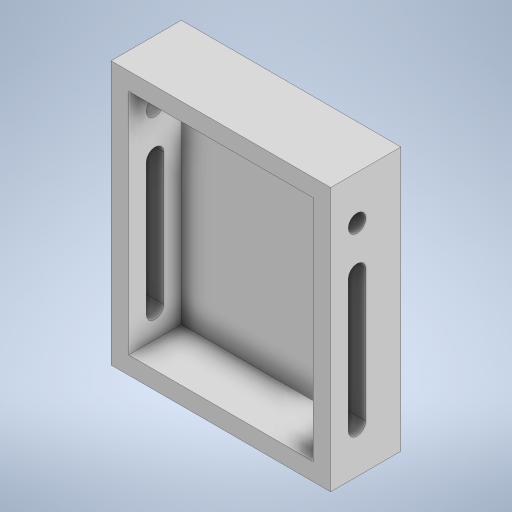
# Autodesk Inventor part: podstawa
Saved by Autodesk Inventor 2024 (Build 280153000, 153)
## iProperties
Created: 2024-09-19
Part Number: podstawa
Material: Ogólny
Document SubType Name: Modeling
Designer: JEDEN
Density: 1 g/cm^3
Appearance: Domyślna
Author: JEDEN
Autodesk Inventor part; units mm, degrees
ref_plane "YZ Plane" through (0, 0, 0) normal (1, 0, 0) x (0, 1, 0)
ref_plane "XZ Plane" through (0, 0, 0) normal (0, 1, 0) x (-1, 0, 0)
ref_plane "XY Plane" through (0, 0, 0) normal (0, 0, 1) x (1, 0, 0)
sketch "Szkic1" plane through (0, 0, 0) normal (0, 0, 1) x (1, 0, 0)
  line L0 (107.302, 11.5082) -> (232.302, 11.5082)
  line L1 (232.302, 11.5082) -> (232.302, -288.4918)
  line L2 (232.302, -288.4918) -> (107.302, -288.4918)
  line L3 (107.302, -288.4918) -> (107.302, 11.5082)
  point P0 (0, 0)
  dimension "d0" = 125
  dimension "d1" = 300
  constraints: 8 end point, 2 parallel, 1 horizontal, 1 perpendicular
  measures "d0" distance of L1.end L2.end
  measures "d1" distance of L0.end L1.end
extrude "Wyciągnięcie proste1" add sketch "Szkic1" along normal blind 20
sketch "Szkic2" plane through (0, 0, 20) normal (0, 0, 1) x (1, 0, 0)
  line L0 (232.302, 11.5082) -> (107.302, 11.5082) projected
  line L1 (107.302, -288.4918) -> (232.302, -288.4918) projected
  line L2 (107.302, 11.5082) -> (127.302, 11.5082)
  line L3 (127.302, 11.5082) -> (127.302, -288.4918)
  line L4 (127.302, -288.4918) -> (107.302, -288.4918)
  line L5 (107.302, -288.4918) -> (107.302, 11.5082)
  line L6 (232.302, -288.4918) -> (232.302, 11.5082) projected
  line L7 (107.302, 11.5082) -> (232.302, 11.5082)
  line L8 (232.302, 11.5082) -> (232.302, -8.4918)
  line L9 (232.302, -8.4918) -> (107.302, -8.4918)
  line L10 (107.302, -8.4918) -> (107.302, 11.5082)
  line L11 (107.302, -288.4918) -> (232.302, -288.4918)
  line L12 (232.302, -288.4918) -> (232.302, -268.4918)
  line L13 (232.302, -268.4918) -> (107.302, -268.4918)
  line L14 (107.302, -268.4918) -> (107.302, -288.4918)
  point P0 (0, 0)
  point P1 (127.302, -8.4918)
  point P2 (127.302, -268.4918)
  dimension "d4" = 20
  dimension "d5" = 20
  dimension "d8" = 20
  constraints: 24 end point, 6 parallel, 3 horizontal, 3 perpendicular, 3 point on line
  measures "d4" distance of L3.end L4.end
  measures "d5" distance of L7.end L8.end
  measures "d8" distance of L12.end L11.end
extrude "Wyciągnięcie proste2" add sketch "Szkic2" along normal blind 60 contours L6 L9 L3 L0 | L3 L9 L5 L0 | L3 L13 L5 L9 | L6 L1 L3 L13 | L3 L1 L5 L13
sketch "Szkic3" plane through (107.302, -288.4918, 0) normal (-1, 0, 0) x (0, 0, 1)
  line L0 (0, 300) -> (80, 300) projected
  line L1 (0, 0) -> (80, 0) projected
  line L2 (80, 300) -> (50, 300)
  line L3 (50, 300) -> (50, 0)
  line L4 (50, 0) -> (80, 0)
  line L5 (80, 0) -> (80, 300)
  circle A0 centre (50, 250) radius 10
  circle A1 centre (50, 200) radius 10
  circle A2 centre (50, 50) radius 10
  line L6 (50, 200) -> (50, 50) construction
  line L7 (40, 200) -> (40, 50)
  line L8 (60, 50) -> (60, 200)
  arc A3 (60, 200) -> (40, 200) centre (50, 200) ccw
  arc A4 (40, 50) -> (60, 50) centre (50, 50) ccw
  point P0 (0, 288.4918)
  point P1 (65, 300)
  point P2 (65, 0)
  point P3 (50, 125)
  point P4 (60, 200)
  dimension "d9" = 30
  dimension "d10" = 50
  dimension "d11" = 50
  dimension "d12" = 100
  dimension "d13" = 20
  dimension "d14" = 20
  dimension "d15" = 20
  constraints: 16 end point, 5 centre point, 4 point on circle, 4 point on line, 4 tangent, 3 coincident, 3 midpoint, 3 parallel, 1 collinear, 1 concentric, 1 horizontal, 1 perpendicular
  measures "d9" distance of L4.end L3.end
  measures "d10" vertical distance of point (65, 300) point (50, 250)
  measures "d11" vertical distance of point (65, 0) point (50, 50)
  measures "d12" distance from line of L0 point (50, 200)
  measures "d13" diameter of A0
  measures "d14" diameter of A1
  measures "d15" diameter of A2
extrude "Wyciągnięcie proste3" cut sketch "Szkic3" against normal through all contours A0 L3 | L3 A0 | A1 L3 | L3 A1 | A2 L3 | L3 A2 | A1 L8 A2 L3 | L3 A2 L7 A1
mirror "Odbij1" about plane through (232.302, -288.4918, 0) normal (1, 0, 0)
